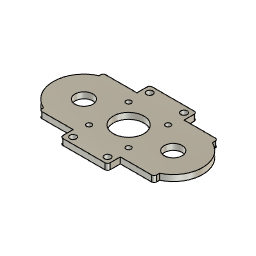
Gearbox Housing - Motor Mount Plane v3 (Autodesk Fusion 360 design; units mm, degrees)
Autodesk Fusion 360 part; units mm, degrees
sketch "Motor Mount" plane through (0, 0, 0) normal (0, 0, 1) x (1, 0, 0)
  line L0 (0, 0) -> (33, 0)
  line L1 (35, 2) -> (35, 10)
  line L2 (61.5, 55.7123) -> (61.5, 58)
  line L3 (-2, 10) -> (-2, 2)
  arc A0 (61.5, 14.2877) -> (61.5, 55.7123) centre (51.5, 35) ccw
  line L4 (61.5, 12) -> (61.5, 14.2877)
  arc A1 (-28.5, 56.7624) -> (-28.5, 13.2376) centre (-18.5, 35) ccw
  arc A2 (61.5, 58) -> (59.5, 60) centre (59.5, 58) ccw
  arc A3 (-2, 2) -> (0, 0) centre (0, 2) ccw
  line L5 (33, 70) -> (0, 70)
  line L6 (-26.5, 10) -> (-2, 10)
  line L7 (-28.5, 58) -> (-28.5, 56.7624)
  line L8 (-2, 60) -> (-26.5, 60)
  arc A4 (0, 70) -> (-2, 68) centre (0, 68) ccw
  arc A5 (59.5, 10) -> (61.5, 12) centre (59.5, 12) ccw
  line L9 (59.5, 60) -> (35, 60)
  line L10 (-2, 68) -> (-2, 60)
  arc A6 (35, 68) -> (33, 70) centre (33, 68) ccw
  arc A7 (-26.5, 60) -> (-28.5, 58) centre (-26.5, 58) ccw
  arc A8 (-28.5, 12) -> (-26.5, 10) centre (-26.5, 12) ccw
  line L11 (35, 60) -> (35, 68)
  arc A9 (33, 0) -> (35, 2) centre (33, 2) ccw
  line L12 (35, 10) -> (59.5, 10)
  line L13 (-28.5, 13.2376) -> (-28.5, 12)
  circle A10 centre (30, 65) radius 2.5
  circle A11 centre (30, 5) radius 2.5
  circle A12 centre (3, 5) radius 2.5
  circle A13 centre (-18.5, 35) radius 7
  circle A14 centre (1, 50.5) radius 2
  circle A15 centre (32, 50.5) radius 2
  circle A16 centre (51.5, 35) radius 7
  circle A17 centre (1, 19.5) radius 2
  circle A18 centre (3, 65) radius 2.5
  circle A19 centre (16.5, 35) radius 12
  circle A20 centre (32, 19.5) radius 2
extrude "Face1" add sketch "Motor Mount" along normal blind 4.75
